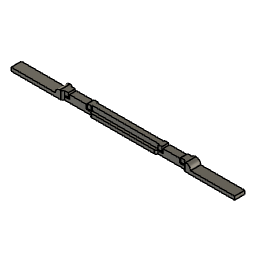
Din Rail Holder (Autodesk Fusion 360 design; units mm, degrees)
part number: DIn Rail Holder
Autodesk Fusion 360 part; units mm, degrees
sketch "Sketch1" plane through (0, 0, 0) normal (0, 1, 0) x (-1, 0, 0)
  line L0 (0, 0) -> (-54.91, 0)
  line L1 (0, 0) -> (54.91, 0)
  line L2 (-50.91, -6) -> (-54.91, -6)
  line L3 (-56.61, -1.5) -> (-56.61, -7.7)
  line L4 (-56.61, -7.7) -> (-50.91, -7.7)
  line L5 (-82.91, -6) -> (-86.91, -6)
  line L6 (-81.21, -1.5) -> (-56.61, -1.5)
  line L7 (-86.91, -6) -> (-86.91, -7.7)
  line L8 (-82.91, 0) -> (-82.91, -6)
  line L9 (-81.21, -7.7) -> (-81.21, -1.5)
  line L10 (-50.91, -7.7) -> (-50.91, -6)
  line L11 (-54.91, -6) -> (-54.91, 0)
  line L12 (-86.91, -7.7) -> (-81.21, -7.7)
  line L13 (54.91, -6) -> (50.91, -6)
  line L14 (50.91, -7.7) -> (56.61, -7.7)
  line L15 (86.91, -7.7) -> (86.91, -6)
  line L16 (81.21, -1.5) -> (81.21, -7.7)
  line L17 (82.91, -6) -> (82.91, 0)
  line L18 (56.61, -7.7) -> (56.61, -1.5)
  line L19 (86.91, -6) -> (82.91, -6)
  line L20 (56.61, -1.5) -> (81.21, -1.5)
  line L21 (54.91, 0) -> (54.91, -6)
  line L22 (81.21, -7.7) -> (86.91, -7.7)
  line L23 (50.91, -6) -> (50.91, -7.7)
  line L24 (-82.91, 0) -> (-88.66, 0)
  line L25 (-88.66, 0) -> (-88.66, -12)
  line L26 (-54.91, 0) -> (-49.16, 0)
  line L27 (-49.16, 0) -> (-49.16, -12)
  line L28 (82.91, 0) -> (88.66, 0)
  line L29 (54.91, 0) -> (49.16, 0)
  line L30 (49.16, 0) -> (49.16, -12)
  line L31 (88.66, 0) -> (88.66, -12)
  line L32 (88.66, 0) -> (99.66, 0)
  line L33 (99.66, 0) -> (99.66, -12)
  line L34 (-88.66, 0) -> (-99.66, 0)
  line L35 (-99.66, 0) -> (-99.66, -12)
  line L36 (99.66, -12) -> (164.66, -12)
  line L37 (164.66, -12) -> (164.66, -7)
  line L38 (164.66, -7) -> (99.66, -7)
  line L39 (99.66, -7) -> (99.66, -12)
  line L40 (-99.66, -12) -> (-164.66, -12)
  line L41 (-164.66, -12) -> (-164.66, -7)
  line L42 (-164.66, -7) -> (-99.66, -7)
  line L43 (-99.66, -7) -> (-99.66, -12)
  line L44 (-49.16, -12) -> (-49.16, -7)
  line L45 (49.16, -7) -> (49.16, -12)
  line L46 (49.16, -12) -> (49.16, -7)
  line L47 (-49.16, -7) -> (-49.16, -12)
  line L48 (-99.66, -12) -> (99.66, -12)
  line L49 (49.16, -12) -> (-49.16, -12)
  line L50 (-49.16, -12) -> (-49.16, -7)
  line L51 (-49.16, -7) -> (49.16, -7)
  line L52 (49.16, -7) -> (49.16, -12)
  dimension "d1" = 54.91
  dimension "d2" = 54.91
  dimension "d5" = 5.75
  dimension "d6" = 12
  dimension "d7" = 5.75
  dimension "d8" = 12
  dimension "d9" = 5.75
  dimension "d10" = 5.75
  dimension "d11" = 12
  dimension "d12" = 12
  dimension "d13" = 11
  dimension "d14" = 12
  dimension "d15" = 11
  dimension "d16" = 12
  dimension "d17" = 65
  dimension "d18" = 5
  dimension "d19" = 65
  dimension "d20" = 5
  dimension "d37" = 5
  constraint coincident L0.start L1.start
  constraint horizontal L0
  constraint parallel L0 L1
  constraint perpendicular L8 L24
  constraint perpendicular L24 L25
  constraint perpendicular L11 L26
  constraint perpendicular L0 L27
  constraint perpendicular L17 L28
  constraint perpendicular L21 L29
  constraint perpendicular L1 L30
  constraint perpendicular L28 L31
  constraint perpendicular L31 L32
  constraint perpendicular L32 L33
  constraint perpendicular L25 L34
  constraint perpendicular L34 L35
  constraint horizontal L36
  constraint vertical L37
  constraint horizontal L38
  constraint vertical L39
  constraint horizontal L40
  constraint vertical L41
  constraint horizontal L42
  constraint vertical L43
  constraint vertical L44
  constraint vertical L45
  constraint vertical L46
  constraint vertical L47
  constraint perpendicular L39 L48
  constraint horizontal L49
  constraint vertical L50
  constraint horizontal L51
  constraint vertical L52
  measures "d1" distance of L0.start L0.end
  measures "d2" distance of L0.start L1.end
  measures "d5" distance of L8.start L24.end
  measures "d6" distance of L24.end L25.end
  measures "d7" distance of L0.end L26.end
  measures "d8" distance of L26.end L27.end
  measures "d9" distance of L17.end L28.end
  measures "d10" distance of L1.end L29.end
  measures "d11" distance of L29.end L30.end
  measures "d12" distance of L28.end L31.end
  measures "d13" distance of L28.end L32.end
  measures "d14" distance of L32.end L33.end
  measures "d15" distance of L24.end L34.end
  measures "d16" distance of L34.end L35.end
  measures "d17" distance of L33.end L36.end
  measures "d18" distance of L33.end L38.end
  measures "d19" distance of L35.end L40.end
  measures "d20" distance of L35.end L42.end
  measures "d37" distance of L30.end L45.start
extrude "Extrude1" add sketch "Sketch1" along normal blind 10 from surface at 2.5 contours L0 L2 L3 L4 L5 L6 L7 L8 L9 L10 L11 L12 L24 L25 L26 L27 L44 L47 L48 L50 | L1 L13 L14 L15 L16 L17 L18 L19 L20 L21 L22 L23 L28 L29 L30 L31 L45 L46 L48 L52 makes body 1 at (-64.81, 2.5, -3.5667) makes body 2 at (73.01, 2.5, -3.5667)
extrude "Extrude2" add sketch "Sketch1" along normal blind 7 from surface at 4 contours L0 L1 L27 L30 L51 bodies 1 2
extrude "Extrude3" add sketch "Sketch1" along normal blind 15 contours L25 L34 L35 L43 L48 | L31 L32 L33 L39 L48 | L35 L40 L41 L42 L43 | L33 L36 L37 L38 L39 bodies 1
fillet "Fillet1" radius 7 1 edges at (99.66, 7.5, 0) on bodies 1
fillet "Fillet2" radius 7 1 edges at (-99.66, 7.5, 0) on bodies 1
fillet "Fillet3" radius 3 2 edges at (-88.66, 15, -6) (88.66, 15, -6) on bodies 1
fillet "Fillet4" radius 3 2 edges at (88.66, 0, -6) (-88.66, 0, -6) on bodies 1
extrude "Extrude4" add sketch "Sketch1" along normal blind 15 contours L27 L30 L44 L45 L46 L47 L48 L49 L50 L51 L52 bodies 1
fillet "Fillet5" radius 3 2 edges at (49.16, 15, -9.5) (-49.16, 15, -9.5) on bodies 1
fillet "Fillet6" radius 3 2 edges at (49.16, 0, -9.5) (-49.16, 0, -9.5) on bodies 1
named bodies: "Din Rail Holder"
